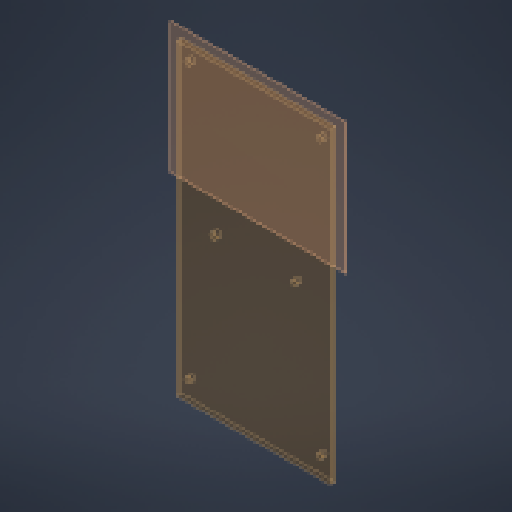
# Autodesk Inventor part: BP_CoverPlateAcrylic
Saved by Autodesk Inventor 2026.1 (Build 301233020, 233B)
## iProperties
Created: 2025-09-13
Part Number: BP_CoverPlateAcrylic
Material: PMMA Plastic
Document SubType Name: Modeling
Designer: atrus
Density: 1.188 g/cm^3
Appearance: Polycarbonate - Smoked
Author: atrus
Autodesk Inventor part; units mm, degrees
ref_plane "YZ Plane" through (0, 0, 0) normal (1, 0, 0) x (0, 1, 0)
ref_plane "XZ Plane" through (0, 0, 0) normal (0, 1, 0) x (-1, 0, 0)
ref_plane "XY Plane" through (0, 0, 0) normal (0, 0, 1) x (1, 0, 0)
ref_plane "Work Plane1" through (0, 0, 0) normal (0, 0, 1) x (1, 0, 0)
sketch "Sketch1" plane through (0, 0, 0) normal (0, 0, 1) x (1, 0, 0)
  line L0 (-10.216, 5.2) -> (85.116, 5.2)
  line L1 (85.116, 5.2) -> (85.116, -186.4)
  line L2 (85.116, -186.4) -> (-10.216, -186.4)
  line L3 (-10.216, -186.4) -> (-10.216, 5.2)
  line L4 (0, 0.2) -> (74.9, 0.2) construction
  line L5 (0, 0.2) -> (0, -6.8)
  line L6 (-8.95, -53) -> (-8.95, -6.8)
  line L7 (-8.95, -6.8) -> (0, -6.8)
  line L8 (-10.416, 5.4) -> (85.316, 5.4)
  circle A0 centre (78.4, -174.4) radius 1.9
  circle A1 centre (-3.5, -174.4) radius 1.9
  line L9 (85.316, -186.6) -> (85.316, -110.8)
  line L10 (85.316, -110.8) -> (74.9, -110.8)
  line L11 (74.9, -110.8) -> (74.9, -124.8)
  line L12 (74.9, -124.8) -> (83.85, -124.8)
  line L13 (83.85, -124.8) -> (83.85, -170.9)
  line L14 (83.85, -170.9) -> (74.9, -170.9)
  line L15 (74.9, -170.9) -> (74.9, -177.9)
  line L16 (0, -177.9) -> (74.9, -177.9)
  line L17 (0, -170.9) -> (0, -177.9)
  line L18 (0, -170.9) -> (-8.95, -170.9)
  line L19 (-8.95, -170.9) -> (-8.95, -124.8)
  line L20 (-8.95, -124.8) -> (0, -124.8)
  line L21 (0, -110.8) -> (0, -124.8)
  line L22 (0, -110.8) -> (-10.416, -110.8)
  line L23 (-10.416, -110.8) -> (-10.416, -186.6)
  line L24 (-10.416, -186.6) -> (85.316, -186.6)
  circle A2 centre (-3.5, -3.3) radius 1.9
  circle A3 centre (78.4, -3.3) radius 1.9
  line L25 (-10.416, 5.4) -> (-10.416, -67)
  line L26 (-10.416, -67) -> (0, -67)
  line L27 (0, -53) -> (0, -67)
  line L28 (0, -53) -> (-8.95, -53)
  line L29 (-8.95, -53) -> (-8.95, -6.8)
  line L30 (-8.95, -6.8) -> (0, -6.8)
  line L31 (0, 0.2) -> (0, -6.8)
  line L32 (0, 0.2) -> (74.9, 0.2)
  line L33 (74.9, -6.8) -> (74.9, 0.2)
  line L34 (74.9, -6.8) -> (83.85, -6.8)
  line L35 (83.85, -6.8) -> (83.85, -53)
  line L36 (83.85, -53) -> (74.9, -53)
  line L37 (74.9, -67) -> (74.9, -53)
  line L38 (74.9, -67) -> (85.316, -67)
  line L39 (85.316, -67) -> (85.316, 5.4)
  line L40 (85.316, 5.4) -> (-10.416, 5.4)
  point P0 (0, 0)
extrude "Extrusion1" add sketch "Sketch1" along normal blind 3 contours L0 L1 L38 L37 L36 L35 L34 L33 L32 L5 L7 L6 L28 L27 L26 L3 | L26 L27 L28 L6 L7 L5 L32 L33 L34 L35 L36 L37 L38 L1 L10 L11 L12 L13 L14 L15 L16 L17 L18 L19 L20 L21 L22 L3 | L22 L21 L20 L19 L18 L17 L16 L15 L14 L13 L12 L11 L10 L1 L2 L3 | A0 | A1 | A2 | A3
sketch "Sketch2" plane through (0, 0, 3) normal (0, 0, 1) x (1, 0, 0)
  circle A0 centre (78.4, -3.3) radius 1.9 projected
  circle A1 centre (-3.5, -3.3) radius 1.9 projected
  circle A2 centre (12.45, -88.9) radius 1.9 projected
  circle A3 centre (62.45, -88.9) radius 1.9 projected
  circle A4 centre (78.4, -174.4) radius 1.9 projected
  circle A5 centre (-3.5, -174.4) radius 1.9 projected
  point P0 (0, 0)
extrude "Extrusion2" cut sketch "Sketch2" against normal blind 3
body "Solid1"
